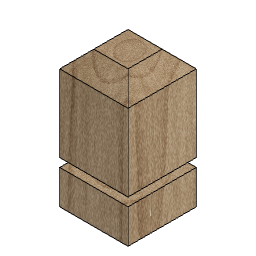
Pawn (Autodesk Fusion 360 design; units mm, degrees)
Autodesk Fusion 360 part; units mm, degrees
note: some values were not read from the file. Chosen so that the rebuilt part matches the saved one: that a step has no effect.
sketch "Sketch1" plane through (0, 0, 0) normal (0, 0, 1) x (1, 0, 0)
  line L0 (-12.7, 12.7) -> (12.7, 12.7)
  line L1 (12.7, 12.7) -> (12.7, -12.7)
  line L2 (12.7, -12.7) -> (-12.7, -12.7)
  line L3 (-12.7, -12.7) -> (-12.7, 12.7)
  constraint horizontal L0
  constraint vertical L1
  constraint horizontal L2
  constraint vertical L3
extrude "Extrude1" add sketch "Sketch1" along normal blind 50.8
sketch "Sketch2" plane through (0, -12.7, 0) normal (0, -1, 0) x (1, 0, 0)
  line L0 (-12.7, 0) -> (12.7, 0)
  line L1 (12.7, 0) -> (12.7, 50.8)
  line L2 (12.7, 50.8) -> (-12.7, 50.8)
  line L3 (-12.7, 50.8) -> (-12.7, 0)
  line L4 (-12.7, 12.7) -> (12.7, 12.7)
  line L5 (12.7, 12.7) -> (12.7, 15.875)
  line L6 (12.7, 15.875) -> (-12.7, 15.875)
  line L7 (-12.7, 15.875) -> (-12.7, 12.7)
  dimension "d4" = 3.175
  constraint coincident L3 L4.start
  constraint horizontal L4
  constraint vertical L5
  constraint horizontal L6
  constraint vertical L7
  measures "d4" distance of L4.start L6.end
sketch "Sketch3" plane through (12.7, 0, 0) normal (1, 0, 0) x (0, 1, 0)
  line L0 (-12.7, 0) -> (12.7, 0)
  line L1 (12.7, 0) -> (12.7, 50.8)
  line L2 (12.7, 50.8) -> (-12.7, 50.8)
  line L3 (-12.7, 50.8) -> (-12.7, 0)
  line L4 (0, 12.7) -> (-12.7, 12.7)
  line L5 (0, 12.7) -> (12.7, 12.7)
  line L6 (-12.7, 12.7) -> (12.7, 12.7)
  line L7 (12.7, 12.7) -> (12.7, 15.875)
  line L8 (12.7, 15.875) -> (-12.7, 15.875)
  line L9 (-12.7, 15.875) -> (-12.7, 12.7)
  dimension "d5" = 3.175
  constraint coincident L3 L4.end
  constraint perpendicular L3 L4
  constraint coincident L1 L5.end
  constraint perpendicular L1 L5
  constraint horizontal L6
  constraint vertical L7
  constraint horizontal L8
  constraint vertical L9
  measures "d5" distance of L4.end L8.end
sketch "Sketch4" plane through (-12.7, 0, 0) normal (-1, 0, 0) x (0, -1, 0)
  line L0 (-12.7, 0) -> (12.7, 0)
  line L1 (12.7, 0) -> (12.7, 50.8)
  line L2 (12.7, 50.8) -> (-12.7, 50.8)
  line L3 (-12.7, 50.8) -> (-12.7, 0)
  line L4 (-12.7, 12.7) -> (12.7, 12.7)
  line L5 (12.7, 12.7) -> (12.7, 15.875)
  line L6 (12.7, 15.875) -> (-12.7, 15.875)
  line L7 (-12.7, 15.875) -> (-12.7, 12.7)
  dimension "d6" = 3.175
  constraint horizontal L4
  constraint vertical L5
  constraint horizontal L6
  constraint vertical L7
  constraint coincident L1 L5.end
  constraint coincident L3 L4.start
  measures "d6" distance of L4.start L6.end
extrude "Extrude2" cut sketch "Sketch4" against normal blind 3.175 contours L1 L3 L4 L5 L6 L7
extrude "Extrude3" cut sketch "Sketch2" against normal blind 3.175 contours L1 L3 L4 L5 L6 L7
extrude "Extrude4" cut sketch "Sketch3" against normal blind 3.175 contours L1 L3 L4 L5 L6 L7 L8 L9
draft "Draft1" [no effect]
chamfer "Chamfer1" distance 6.35 angle 45 4 edges at (0, -12.7, 50.8) (-12.7, 0, 50.8) (0, 12.7, 50.8) (12.7, 0, 50.8)
equation "d4 = ( 1 / 8 ) * 1 in"
equation "d5 = ( 1 / 8 ) * 1 in"
equation "d6 = ( 1 / 8 ) * 1 in"
equation "d7 = ( -1 / 8 ) * 1 in"
equation "d9 = ( -1 / 8 ) * 1 in"
equation "d11 = ( -1 / 8 ) * 1 in"
equation "d15 = ( 1 / 4 ) * 1 in"
